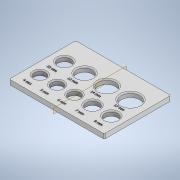
# Autodesk Inventor part: mmHexSocketSetOf9
Saved by Autodesk Inventor 2020.3 (Build 243373000, 373)
## iProperties
Created: 2020-03-13
Part Number: mmHexSocketSetOf9
Material: Generic
Document SubType Name: Modeling
Designer: robst
Density: 1 g/cm^3
Appearance: Default
Author: robst
Autodesk Inventor part; units mm, degrees
(part 1 of 2)
ref_plane "XZ Plane" through (0, 0, 0) normal (0, 1, 0) x (-1, 0, 0)
ref_plane "XY Plane" through (0, 0, 0) normal (0, 0, 1) x (1, 0, 0)
sketch "Sketch1" plane through (0, 0, 0) normal (0, 1, 0) x (-1, 0, 0)
  line L0 (63.5, 44.45) -> (-63.5, 44.45)
  line L1 (-63.5, 44.45) -> (-63.5, -44.45)
  line L2 (-63.5, -44.45) -> (63.5, -44.45)
  line L3 (63.5, -44.45) -> (63.5, 44.45)
  line L4 (63.5, 44.45) -> (-63.5, -44.45) construction
  line L5 (-63.5, 44.45) -> (63.5, -44.45) construction
  point P0 (0, 0)
  dimension "d3" = 88.9
  dimension "d13" = 127
  constraints: 12 end point, 2 midpoint, 2 parallel, 1 horizontal, 1 perpendicular
  measures "d3" distance of L2.end L0.start
  measures "d13" distance of L1.end L2.end
extrude "Extrusion1" add sketch "Sketch1" against normal blind 6.35
sketch "Sketch4" plane through (0, 0, 0) normal (0, 1, 0) x (1, 0, 0)
  line L0 (-63.5, -44.45) -> (-63.5, 44.45) construction
  line L1 (-63.5, -19.05) -> (63.5, -19.05) construction
  line L2 (63.5, 44.45) -> (63.5, -44.45) construction
  line L3 (-63.5, -44.45) -> (63.5, -44.45) projected
  circle A0 centre (-47.9975, -19.05) radius 7.62
  circle A1 centre (-24.8751, -19.05) radius 7.62
  circle A2 centre (-1.7526, -19.05) radius 7.62
  circle A3 centre (22.3859, -19.05) radius 8.636
  circle A4 centre (47.5403, -19.05) radius 8.636
  line L4 (-63.5, 12.7) -> (63.5, 12.7) construction
  circle A5 centre (-46.99, 12.7) radius 8.636
  circle A6 centre (-20.0025, 12.7) radius 10.4775
  circle A7 centre (9.779, 12.7) radius 11.43
  circle A8 centre (41.4655, 12.7) radius 12.3825
  point P0 (0, 0)
  dimension "d16" = 25.4
  dimension "hex4mmHole" = 15.24
  dimension "gap0" = 7.8825
  dimension "hex5mmHole" = 15.24
  dimension "gap1" = 23.1225
  dimension "hex6mmHole" = 15.24
  dimension "gap2" = 23.1225
  dimension "gap3" = 24.1385
  dimension "gap4" = 25.1545
  dimension "hex7mmHole" = 17.272
  dimension "hex8mmHole" = 17.272
  dimension "d27" = 7.3237
  dimension "frontToBackRowGap" = 31.75
  dimension "gap5" = 7.874
  dimension "hex10mmHole" = 17.272
  dimension "hex12mmHole" = 20.955
  dimension "gap6" = 26.9875
  dimension "hex14mmHole" = 22.86
  dimension "gap7" = 29.7815
  dimension "hex17mmHole" = 24.765
  dimension "gap8" = 31.6865
  dimension "d37" = 9.652
  constraints: 13 point on line, 9 centre point, 4 end point, 1 horizontal, 1 perpendicular
  measures "d16" distance between parallel lines of L1 L3
  measures "hex4mmHole" diameter of A0
  measures "gap0" distance edge to line of A0 L0
  measures "hex5mmHole" diameter of A1
  measures "gap1" distance of A1.centre A0.centre
  measures "hex6mmHole" diameter of A2
  measures "gap2" distance of A2.centre A1.centre
  measures "gap3" distance of A3.centre A2.centre
  measures "gap4" distance of A4.centre A3.centre
  measures "hex7mmHole" diameter of A3
  measures "hex8mmHole" diameter of A4
  measures "d27" distance edge to line of A4 L2
  measures "frontToBackRowGap" distance between parallel lines of L4 L1
  measures "gap5" distance edge to line of A5 L0
  measures "hex10mmHole" diameter of A5
  measures "hex12mmHole" diameter of A6
  measures "gap6" distance of A6.centre A5.centre
  measures "hex14mmHole" diameter of A7
  measures "gap7" distance of A7.centre A6.centre
  measures "hex17mmHole" diameter of A8
  measures "gap8" distance of A8.centre A7.centre
  measures "d37" distance edge to line of A8 L2
extrude "Extrusion3" cut sketch "Sketch4" against normal through all
sketch "Sketch7" plane through (0, 0, 0) normal (0, 1, 0) x (1, 0, 0)
  circle A0 centre (-47.9975, -19.05) radius 7.62 construction
  line L0 (63.5, -44.45) -> (-63.5, -44.45) construction
  line L1 (-55.6175, -35.6779) -> (-40.3775, -35.6779) construction
  line L2 (-32.4951, -35.6779) -> (-17.2551, -35.6779) construction
  line L3 (-9.3726, -35.6779) -> (5.8674, -35.6779) construction
  line L4 (13.7499, -35.6779) -> (30.7679, -35.6779) construction
  line L5 (38.6503, -35.6779) -> (55.6683, -35.6779) construction
  line L6 (-55.626, -3.81) -> (-38.354, -3.81) construction
  line L7 (-30.48, -3.81) -> (-7.62, -3.81) construction
  line L8 (0.254, -3.81) -> (23.114, -3.81) construction
  line L9 (30.988, -3.81) -> (55.626, -3.81) construction
  line L10 (-51.5027, -5.334) -> (-52.9897, -5.334)
  line L11 (-52.9897, -5.334) -> (-52.9897, -5.0228)
  line L12 (-52.9897, -5.0228) -> (-52.4364, -5.0228)
  line L13 (-52.4364, -5.0228) -> (-52.4364, -2.9801)
  line L14 (-52.4364, -2.9801) -> (-52.9897, -2.9801)
  line L15 (-52.9897, -2.9801) -> (-52.9897, -2.701)
  spline S0 degree 2 poles (-52.9897, -2.701) (-52.676, -2.701) (-52.3796, -2.5231) (-52.3598, -2.2761) knots 0 0 0 1 2 2 2
  line L16 (-52.3598, -2.2761) -> (-52.0437, -2.2761)
  line L17 (-52.0437, -2.2761) -> (-52.0437, -5.0228)
  line L18 (-52.0437, -5.0228) -> (-51.5027, -5.0228)
  line L19 (-51.5027, -5.0228) -> (-51.5027, -5.334)
  spline S1 degree 2 poles (-49.0451, -3.81) (-49.0451, -4.63) (-49.5218, -5.3982) (-50.0182, -5.3982) knots 0 0 0 1 2 2 2
  spline S2 degree 2 poles (-50.0182, -5.3982) (-50.5221, -5.3982) (-50.9939, -4.6152) (-50.9939, -3.8125) knots 0 0 0 1 2 2 2
  spline S3 degree 2 poles (-50.9939, -3.8125) (-50.9939, -2.9875) (-50.5172, -2.2242) (-50.0182, -2.2242) knots 0 0 0 1 2 2 2
  spline S4 degree 2 poles (-50.0182, -2.2242) (-49.5168, -2.2242) (-49.0451, -3.0147) (-49.0451, -3.81) knots 0 0 0 1 2 2 2
  spline S5 degree 2 poles (-49.5687, -4.7387) (-49.5094, -4.5881) (-49.46, -4.1237) (-49.46, -3.81) knots 0 0 0 1 2 2 2
  spline S6 degree 2 poles (-49.46, -3.81) (-49.46, -3.4963) (-49.5094, -3.0344) (-49.5712, -2.8788) knots 0 0 0 1 2 2 2
  spline S7 degree 2 poles (-49.5712, -2.8788) (-49.6329, -2.7232) (-49.8478, -2.5626) (-50.0182, -2.5626) knots 0 0 0 1 2 2 2
  spline S8 degree 2 poles (-50.0182, -2.5626) (-50.1887, -2.5626) (-50.4085, -2.7232) (-50.4727, -2.8837) knots 0 0 0 1 2 2 2
  spline S9 degree 2 poles (-50.4727, -2.8837) (-50.5345, -3.0394) (-50.5789, -3.5136) (-50.5789, -3.8125) knots 0 0 0 1 2 2 2
  spline S10 degree 2 poles (-50.5789, -3.8125) (-50.5789, -4.1336) (-50.5394, -4.5634) (-50.4752, -4.7313) knots 0 0 0 1 2 2 2
  spline S11 degree 2 poles (-50.4752, -4.7313) (-50.4159, -4.8894) (-50.1961, -5.0598) (-50.0182, -5.0598) knots 0 0 0 1 2 2 2
  spline S12 degree 2 poles (-50.0182, -5.0598) (-49.8503, -5.0598) (-49.6304, -4.8993) (-49.5687, -4.7387) knots 0 0 0 1 2 2 2
  line L20 (-44.6954, -5.334) -> (-44.6954, -4.0101)
  spline S13 degree 2 poles (-44.6954, -4.0101) (-44.6954, -3.852) (-44.7201, -3.5828) (-44.7596, -3.5087) knots 0 0 0 1 2 2 2
  spline S14 degree 2 poles (-44.7596, -3.5087) (-44.7991, -3.4271) (-44.9498, -3.3481) (-45.0807, -3.3481) knots 0 0 0 1 2 2 2
  spline S15 degree 2 poles (-45.0807, -3.3481) (-45.1992, -3.3481) (-45.4709, -3.4938) (-45.6142, -3.6322) knots 0 0 0 1 2 2 2
  spline S16 degree 2 poles (-45.6142, -3.6322) (-45.6117, -3.6667) (-45.6068, -3.7631) (-45.6068, -3.8273) knots 0 0 0 1 2 2 2
  line L21 (-45.6068, -3.8273) -> (-45.6068, -5.334)
  line L22 (-45.6068, -5.334) -> (-45.9921, -5.334)
  line L23 (-45.9921, -5.334) -> (-45.9921, -4.0101)
  spline S17 degree 2 poles (-45.9921, -4.0101) (-45.9921, -3.852) (-46.0168, -3.5828) (-46.0563, -3.5087) knots 0 0 0 1 2 2 2
  spline S18 degree 2 poles (-46.0563, -3.5087) (-46.0959, -3.4271) (-46.2465, -3.3481) (-46.3774, -3.3481) knots 0 0 0 1 2 2 2
  spline S19 degree 2 poles (-46.3774, -3.3481) (-46.5009, -3.3481) (-46.7751, -3.5037) (-46.9035, -3.6247) knots 0 0 0 1 2 2 2
  line L24 (-46.9035, -3.6247) -> (-46.9035, -5.334)
  line L25 (-46.9035, -5.334) -> (-47.2889, -5.334)
  line L26 (-47.2889, -5.334) -> (-47.2889, -3.0468)
  line L27 (-47.2889, -3.0468) -> (-46.9035, -3.0468)
  line L28 (-46.9035, -3.0468) -> (-46.9035, -3.2987)
  spline S20 degree 2 poles (-46.9035, -3.2987) (-46.7529, -3.148) (-46.4565, -2.9825) (-46.2786, -2.9825) knots 0 0 0 1 2 2 2
  spline S21 degree 2 poles (-46.2786, -2.9825) (-46.0761, -2.9825) (-45.7624, -3.1678) (-45.6809, -3.3777) knots 0 0 0 1 2 2 2
  spline S22 degree 2 poles (-45.6809, -3.3777) (-45.5055, -3.1826) (-45.1745, -2.9825) (-44.9819, -2.9825) knots 0 0 0 1 2 2 2
  spline S23 degree 2 poles (-44.9819, -2.9825) (-44.8337, -2.9825) (-44.5916, -3.0739) (-44.5027, -3.1777) knots 0 0 0 1 2 2 2
  spline S24 degree 2 poles (-44.5027, -3.1777) (-44.4113, -3.2814) (-44.31, -3.5926) (-44.31, -3.8273) knots 0 0 0 1 2 2 2
  line L29 (-44.31, -3.8273) -> (-44.31, -5.334)
  line L30 (-44.31, -5.334) -> (-44.6954, -5.334)
  line L31 (-41.1756, -5.334) -> (-41.1756, -4.0101)
  spline S25 degree 2 poles (-41.1756, -4.0101) (-41.1756, -3.852) (-41.2003, -3.5828) (-41.2398, -3.5087) knots 0 0 0 1 2 2 2
  spline S26 degree 2 poles (-41.2398, -3.5087) (-41.2793, -3.4271) (-41.43, -3.3481) (-41.5609, -3.3481) knots 0 0 0 1 2 2 2
  spline S27 degree 2 poles (-41.5609, -3.3481) (-41.6795, -3.3481) (-41.9512, -3.4938) (-42.0944, -3.6322) knots 0 0 0 1 2 2 2
  spline S28 degree 2 poles (-42.0944, -3.6322) (-42.092, -3.6667) (-42.087, -3.7631) (-42.087, -3.8273) knots 0 0 0 1 2 2 2
  line L32 (-42.087, -3.8273) -> (-42.087, -5.334)
  line L33 (-42.087, -5.334) -> (-42.4723, -5.334)
  line L34 (-42.4723, -5.334) -> (-42.4723, -4.0101)
  spline S29 degree 2 poles (-42.4723, -4.0101) (-42.4723, -3.852) (-42.497, -3.5828) (-42.5366, -3.5087) knots 0 0 0 1 2 2 2
  spline S30 degree 2 poles (-42.5366, -3.5087) (-42.5761, -3.4271) (-42.7268, -3.3481) (-42.8577, -3.3481) knots 0 0 0 1 2 2 2
  spline S31 degree 2 poles (-42.8577, -3.3481) (-42.9812, -3.3481) (-43.2553, -3.5037) (-43.3838, -3.6247) knots 0 0 0 1 2 2 2
  line L35 (-43.3838, -3.6247) -> (-43.3838, -5.334)
  line L36 (-43.3838, -5.334) -> (-43.7691, -5.334)
  line L37 (-43.7691, -5.334) -> (-43.7691, -3.0468)
  line L38 (-43.7691, -3.0468) -> (-43.3838, -3.0468)
  line L39 (-43.3838, -3.0468) -> (-43.3838, -3.2987)
  spline S32 degree 2 poles (-43.3838, -3.2987) (-43.2331, -3.148) (-42.9367, -2.9825) (-42.7589, -2.9825) knots 0 0 0 1 2 2 2
  spline S33 degree 2 poles (-42.7589, -2.9825) (-42.5563, -2.9825) (-42.2426, -3.1678) (-42.1611, -3.3777) knots 0 0 0 1 2 2 2
  spline S34 degree 2 poles (-42.1611, -3.3777) (-41.9857, -3.1826) (-41.6548, -2.9825) (-41.4621, -2.9825) knots 0 0 0 1 2 2 2
  spline S35 degree 2 poles (-41.4621, -2.9825) (-41.3139, -2.9825) (-41.0718, -3.0739) (-40.9829, -3.1777) knots 0 0 0 1 2 2 2
  spline S36 degree 2 poles (-40.9829, -3.1777) (-40.8915, -3.2814) (-40.7903, -3.5926) (-40.7903, -3.8273) knots 0 0 0 1 2 2 2
  line L40 (-40.7903, -3.8273) -> (-40.7903, -5.334)
  line L41 (-40.7903, -5.334) -> (-41.1756, -5.334)
  line L42 (-23.5627, -5.334) -> (-25.0497, -5.334)
  line L43 (-25.0497, -5.334) -> (-25.0497, -5.0228)
  line L44 (-25.0497, -5.0228) -> (-24.4964, -5.0228)
  line L45 (-24.4964, -5.0228) -> (-24.4964, -2.9801)
  line L46 (-24.4964, -2.9801) -> (-25.0497, -2.9801)
  line L47 (-25.0497, -2.9801) -> (-25.0497, -2.701)
  spline S37 degree 2 poles (-25.0497, -2.701) (-24.736, -2.701) (-24.4396, -2.5231) (-24.4198, -2.2761) knots 0 0 0 1 2 2 2
  line L48 (-24.4198, -2.2761) -> (-24.1037, -2.2761)
  line L49 (-24.1037, -2.2761) -> (-24.1037, -5.0228)
  line L50 (-24.1037, -5.0228) -> (-23.5627, -5.0228)
  line L51 (-23.5627, -5.0228) -> (-23.5627, -5.334)
  line L52 (-21.1223, -5.334) -> (-23.002, -5.334)
  line L53 (-23.002, -5.334) -> (-23.002, -4.9017)
  spline S38 degree 2 poles (-23.002, -4.9017) (-22.7995, -4.7116) (-22.4389, -4.3583) (-22.266, -4.1682) knots 0 0 0 1 2 2 2
  spline S39 degree 2 poles (-22.266, -4.1682) (-21.9177, -3.7853) (-21.6633, -3.3259) (-21.6633, -3.0813) knots 0 0 0 1 2 2 2
  spline S40 degree 2 poles (-21.6633, -3.0813) (-21.6633, -2.9529) (-21.7423, -2.7602) (-21.8139, -2.6985) knots 0 0 0 1 2 2 2
  spline S41 degree 2 poles (-21.8139, -2.6985) (-21.8856, -2.6367) (-22.0733, -2.575) (-22.1869, -2.575) knots 0 0 0 1 2 2 2
  spline S42 degree 2 poles (-22.1869, -2.575) (-22.2956, -2.575) (-22.5179, -2.6293) (-22.6192, -2.6713) knots 0 0 0 1 2 2 2
  spline S43 degree 2 poles (-22.6192, -2.6713) (-22.7056, -2.7059) (-22.8662, -2.8047) (-22.9156, -2.8393) knots 0 0 0 1 2 2 2
  line L54 (-22.9156, -2.8393) -> (-22.9378, -2.8393)
  line L55 (-22.9378, -2.8393) -> (-22.9378, -2.4046)
  spline S44 degree 2 poles (-22.9378, -2.4046) (-22.8118, -2.3428) (-22.3598, -2.2218) (-22.1573, -2.2218) knots 0 0 0 1 2 2 2
  spline S45 degree 2 poles (-22.1573, -2.2218) (-21.73, -2.2218) (-21.2483, -2.6738) (-21.2483, -3.0591) knots 0 0 0 1 2 2 2
  spline S46 degree 2 poles (-21.2483, -3.0591) (-21.2483, -3.2394) (-21.3323, -3.5408) (-21.4064, -3.6692) knots 0 0 0 1 2 2 2
  spline S47 degree 2 poles (-21.4064, -3.6692) (-21.4805, -3.8026) (-21.6954, -4.0644) (-21.8139, -4.1904) knots 0 0 0 1 2 2 2
  spline S48 degree 2 poles (-21.8139, -4.1904) (-22.0066, -4.4003) (-22.4784, -4.8499) (-22.6192, -4.9808) knots 0 0 0 1 2 2 2
  line L56 (-22.6192, -4.9808) -> (-21.1223, -4.9808)
  line L57 (-21.1223, -4.9808) -> (-21.1223, -5.334)
  line L58 (-16.7554, -5.334) -> (-16.7554, -4.0101)
  spline S49 degree 2 poles (-16.7554, -4.0101) (-16.7554, -3.852) (-16.7801, -3.5828) (-16.8196, -3.5087) knots 0 0 0 1 2 2 2
  spline S50 degree 2 poles (-16.8196, -3.5087) (-16.8591, -3.4271) (-17.0098, -3.3481) (-17.1407, -3.3481) knots 0 0 0 1 2 2 2
  spline S51 degree 2 poles (-17.1407, -3.3481) (-17.2592, -3.3481) (-17.5309, -3.4938) (-17.6742, -3.6322) knots 0 0 0 1 2 2 2
  spline S52 degree 2 poles (-17.6742, -3.6322) (-17.6717, -3.6667) (-17.6668, -3.7631) (-17.6668, -3.8273) knots 0 0 0 1 2 2 2
  line L59 (-17.6668, -3.8273) -> (-17.6668, -5.334)
  line L60 (-17.6668, -5.334) -> (-18.0521, -5.334)
  line L61 (-18.0521, -5.334) -> (-18.0521, -4.0101)
  spline S53 degree 2 poles (-18.0521, -4.0101) (-18.0521, -3.852) (-18.0768, -3.5828) (-18.1163, -3.5087) knots 0 0 0 1 2 2 2
  spline S54 degree 2 poles (-18.1163, -3.5087) (-18.1559, -3.4271) (-18.3065, -3.3481) (-18.4374, -3.3481) knots 0 0 0 1 2 2 2
  spline S55 degree 2 poles (-18.4374, -3.3481) (-18.5609, -3.3481) (-18.8351, -3.5037) (-18.9635, -3.6247) knots 0 0 0 1 2 2 2
  line L62 (-18.9635, -3.6247) -> (-18.9635, -5.334)
  line L63 (-18.9635, -5.334) -> (-19.3489, -5.334)
  line L64 (-19.3489, -5.334) -> (-19.3489, -3.0468)
  line L65 (-19.3489, -3.0468) -> (-18.9635, -3.0468)
  line L66 (-18.9635, -3.0468) -> (-18.9635, -3.2987)
  spline S56 degree 2 poles (-18.9635, -3.2987) (-18.8129, -3.148) (-18.5165, -2.9825) (-18.3386, -2.9825) knots 0 0 0 1 2 2 2
  spline S57 degree 2 poles (-18.3386, -2.9825) (-18.1361, -2.9825) (-17.8224, -3.1678) (-17.7409, -3.3777) knots 0 0 0 1 2 2 2
  spline S58 degree 2 poles (-17.7409, -3.3777) (-17.5655, -3.1826) (-17.2345, -2.9825) (-17.0419, -2.9825) knots 0 0 0 1 2 2 2
  spline S59 degree 2 poles (-17.0419, -2.9825) (-16.8937, -2.9825) (-16.6516, -3.0739) (-16.5627, -3.1777) knots 0 0 0 1 2 2 2
  spline S60 degree 2 poles (-16.5627, -3.1777) (-16.4713, -3.2814) (-16.37, -3.5926) (-16.37, -3.8273) knots 0 0 0 1 2 2 2
  line L67 (-16.37, -3.8273) -> (-16.37, -5.334)
  line L68 (-16.37, -5.334) -> (-16.7554, -5.334)
  line L69 (-13.2356, -5.334) -> (-13.2356, -4.0101)
  spline S61 degree 2 poles (-13.2356, -4.0101) (-13.2356, -3.852) (-13.2603, -3.5828) (-13.2998, -3.5087) knots 0 0 0 1 2 2 2
  spline S62 degree 2 poles (-13.2998, -3.5087) (-13.3393, -3.4271) (-13.49, -3.3481) (-13.6209, -3.3481) knots 0 0 0 1 2 2 2
  spline S63 degree 2 poles (-13.6209, -3.3481) (-13.7395, -3.3481) (-14.0112, -3.4938) (-14.1544, -3.6322) knots 0 0 0 1 2 2 2
  spline S64 degree 2 poles (-14.1544, -3.6322) (-14.152, -3.6667) (-14.147, -3.7631) (-14.147, -3.8273) knots 0 0 0 1 2 2 2
  line L70 (-14.147, -3.8273) -> (-14.147, -5.334)
  line L71 (-14.147, -5.334) -> (-14.5323, -5.334)
  line L72 (-14.5323, -5.334) -> (-14.5323, -4.0101)
  spline S65 degree 2 poles (-14.5323, -4.0101) (-14.5323, -3.852) (-14.557, -3.5828) (-14.5966, -3.5087) knots 0 0 0 1 2 2 2
  spline S66 degree 2 poles (-14.5966, -3.5087) (-14.6361, -3.4271) (-14.7868, -3.3481) (-14.9177, -3.3481) knots 0 0 0 1 2 2 2
  spline S67 degree 2 poles (-14.9177, -3.3481) (-15.0412, -3.3481) (-15.3153, -3.5037) (-15.4438, -3.6247) knots 0 0 0 1 2 2 2
  line L73 (-15.4438, -3.6247) -> (-15.4438, -5.334)
  line L74 (-15.4438, -5.334) -> (-15.8291, -5.334)
  line L75 (-15.8291, -5.334) -> (-15.8291, -3.0468)
  line L76 (-15.8291, -3.0468) -> (-15.4438, -3.0468)
  line L77 (-15.4438, -3.0468) -> (-15.4438, -3.2987)
  spline S68 degree 2 poles (-15.4438, -3.2987) (-15.2931, -3.148) (-14.9967, -2.9825) (-14.8189, -2.9825) knots 0 0 0 1 2 2 2
  spline S69 degree 2 poles (-14.8189, -2.9825) (-14.6163, -2.9825) (-14.3026, -3.1678) (-14.2211, -3.3777) knots 0 0 0 1 2 2 2
  spline S70 degree 2 poles (-14.2211, -3.3777) (-14.0457, -3.1826) (-13.7148, -2.9825) (-13.5221, -2.9825) knots 0 0 0 1 2 2 2
  spline S71 degree 2 poles (-13.5221, -2.9825) (-13.3739, -2.9825) (-13.1318, -3.0739) (-13.0429, -3.1777) knots 0 0 0 1 2 2 2
  spline S72 degree 2 poles (-13.0429, -3.1777) (-12.9515, -3.2814) (-12.8503, -3.5926) (-12.8503, -3.8273) knots 0 0 0 1 2 2 2
  line L78 (-12.8503, -3.8273) -> (-12.8503, -5.334)
  line L79 (-12.8503, -5.334) -> (-13.2356, -5.334)
  line L80 (7.1713, -5.334) -> (5.6843, -5.334)
  line L81 (5.6843, -5.334) -> (5.6843, -5.0228)
  line L82 (5.6843, -5.0228) -> (6.2376, -5.0228)
  line L83 (6.2376, -5.0228) -> (6.2376, -2.9801)
  line L84 (6.2376, -2.9801) -> (5.6843, -2.9801)
  line L85 (5.6843, -2.9801) -> (5.6843, -2.701)
  spline S73 degree 2 poles (5.6843, -2.701) (5.998, -2.701) (6.2944, -2.5231) (6.3142, -2.2761) knots 0 0 0 1 2 2 2
  line L86 (6.3142, -2.2761) -> (6.6303, -2.2761)
  line L87 (6.6303, -2.2761) -> (6.6303, -5.0228)
  line L88 (6.6303, -5.0228) -> (7.1713, -5.0228)
  line L89 (7.1713, -5.0228) -> (7.1713, -5.334)
  line L90 (9.6932, -4.2867) -> (9.3301, -4.2867)
  line L91 (9.3301, -4.2867) -> (9.3301, -5.334)
  line L92 (9.3301, -5.334) -> (8.9373, -5.334)
  line L93 (8.9373, -5.334) -> (8.9373, -4.2867)
  line L94 (8.9373, -4.2867) -> (7.5912, -4.2867)
  line L95 (7.5912, -4.2867) -> (7.5912, -3.8569)
  line L96 (7.5912, -3.8569) -> (8.9546, -2.286)
  line L97 (8.9546, -2.286) -> (9.3301, -2.286)
  line L98 (9.3301, -2.286) -> (9.3301, -3.9582)
  line L99 (9.3301, -3.9582) -> (9.6932, -3.9582)
  line L100 (9.6932, -3.9582) -> (9.6932, -4.2867)
  line L101 (8.9373, -3.9582) -> (8.9373, -2.7677)
  line L102 (8.9373, -2.7677) -> (7.9123, -3.9582)
  line L103 (7.9123, -3.9582) -> (8.9373, -3.9582)
  line L104 (13.9786, -5.334) -> (13.9786, -4.0101)
  spline S74 degree 2 poles (13.9786, -4.0101) (13.9786, -3.852) (13.9539, -3.5828) (13.9144, -3.5087) knots 0 0 0 1 2 2 2
  spline S75 degree 2 poles (13.9144, -3.5087) (13.8749, -3.4271) (13.7242, -3.3481) (13.5933, -3.3481) knots 0 0 0 1 2 2 2
  spline S76 degree 2 poles (13.5933, -3.3481) (13.4748, -3.3481) (13.2031, -3.4938) (13.0598, -3.6322) knots 0 0 0 1 2 2 2
  spline S77 degree 2 poles (13.0598, -3.6322) (13.0623, -3.6667) (13.0672, -3.7631) (13.0672, -3.8273) knots 0 0 0 1 2 2 2
  line L105 (13.0672, -3.8273) -> (13.0672, -5.334)
  line L106 (13.0672, -5.334) -> (12.6819, -5.334)
  line L107 (12.6819, -5.334) -> (12.6819, -4.0101)
  spline S78 degree 2 poles (12.6819, -4.0101) (12.6819, -3.852) (12.6572, -3.5828) (12.6177, -3.5087) knots 0 0 0 1 2 2 2
  spline S79 degree 2 poles (12.6177, -3.5087) (12.5781, -3.4271) (12.4275, -3.3481) (12.2966, -3.3481) knots 0 0 0 1 2 2 2
  spline S80 degree 2 poles (12.2966, -3.3481) (12.1731, -3.3481) (11.8989, -3.5037) (11.7705, -3.6247) knots 0 0 0 1 2 2 2
  line L108 (11.7705, -3.6247) -> (11.7705, -5.334)
  line L109 (11.7705, -5.334) -> (11.3851, -5.334)
  line L110 (11.3851, -5.334) -> (11.3851, -3.0468)
  line L111 (11.3851, -3.0468) -> (11.7705, -3.0468)
  line L112 (11.7705, -3.0468) -> (11.7705, -3.2987)
  spline S81 degree 2 poles (11.7705, -3.2987) (11.9211, -3.148) (12.2175, -2.9825) (12.3954, -2.9825) knots 0 0 0 1 2 2 2
  spline S82 degree 2 poles (12.3954, -2.9825) (12.5979, -2.9825) (12.9116, -3.1678) (12.9931, -3.3777) knots 0 0 0 1 2 2 2
  spline S83 degree 2 poles (12.9931, -3.3777) (13.1685, -3.1826) (13.4995, -2.9825) (13.6921, -2.9825) knots 0 0 0 1 2 2 2
  spline S84 degree 2 poles (13.6921, -2.9825) (13.8403, -2.9825) (14.0824, -3.0739) (14.1713, -3.1777) knots 0 0 0 1 2 2 2
  spline S85 degree 2 poles (14.1713, -3.1777) (14.2627, -3.2814) (14.364, -3.5926) (14.364, -3.8273) knots 0 0 0 1 2 2 2
  line L113 (14.364, -3.8273) -> (14.364, -5.334)
  line L114 (14.364, -5.334) -> (13.9786, -5.334)
  line L115 (17.4984, -5.334) -> (17.4984, -4.0101)
  spline S86 degree 2 poles (17.4984, -4.0101) (17.4984, -3.852) (17.4737, -3.5828) (17.4342, -3.5087) knots 0 0 0 1 2 2 2
  spline S87 degree 2 poles (17.4342, -3.5087) (17.3947, -3.4271) (17.244, -3.3481) (17.1131, -3.3481) knots 0 0 0 1 2 2 2
  spline S88 degree 2 poles (17.1131, -3.3481) (16.9945, -3.3481) (16.7228, -3.4938) (16.5796, -3.6322) knots 0 0 0 1 2 2 2
  spline S89 degree 2 poles (16.5796, -3.6322) (16.582, -3.6667) (16.587, -3.7631) (16.587, -3.8273) knots 0 0 0 1 2 2 2
  line L116 (16.587, -3.8273) -> (16.587, -5.334)
  line L117 (16.587, -5.334) -> (16.2017, -5.334)
  line L118 (16.2017, -5.334) -> (16.2017, -4.0101)
  spline S90 degree 2 poles (16.2017, -4.0101) (16.2017, -3.852) (16.177, -3.5828) (16.1374, -3.5087) knots 0 0 0 1 2 2 2
  spline S91 degree 2 poles (16.1374, -3.5087) (16.0979, -3.4271) (15.9472, -3.3481) (15.8163, -3.3481) knots 0 0 0 1 2 2 2
  spline S92 degree 2 poles (15.8163, -3.3481) (15.6928, -3.3481) (15.4187, -3.5037) (15.2902, -3.6247) knots 0 0 0 1 2 2 2
  line L119 (15.2902, -3.6247) -> (15.2902, -5.334)
  line L120 (15.2902, -5.334) -> (14.9049, -5.334)
  line L121 (14.9049, -5.334) -> (14.9049, -3.0468)
  line L122 (14.9049, -3.0468) -> (15.2902, -3.0468)
  line L123 (15.2902, -3.0468) -> (15.2902, -3.2987)
  spline S93 degree 2 poles (15.2902, -3.2987) (15.4409, -3.148) (15.7373, -2.9825) (15.9151, -2.9825) knots 0 0 0 1 2 2 2
  spline S94 degree 2 poles (15.9151, -2.9825) (16.1177, -2.9825) (16.4314, -3.1678) (16.5129, -3.3777) knots 0 0 0 1 2 2 2
  spline S95 degree 2 poles (16.5129, -3.3777) (16.6883, -3.1826) (17.0192, -2.9825) (17.2119, -2.9825) knots 0 0 0 1 2 2 2
  spline S96 degree 2 poles (17.2119, -2.9825) (17.3601, -2.9825) (17.6022, -3.0739) (17.6911, -3.1777) knots 0 0 0 1 2 2 2
  spline S97 degree 2 poles (17.6911, -3.1777) (17.7825, -3.2814) (17.8837, -3.5926) (17.8837, -3.8273) knots 0 0 0 1 2 2 2
  line L124 (17.8837, -3.8273) -> (17.8837, -5.334)
  line L125 (17.8837, -5.334) -> (17.4984, -5.334)
  line L126 (38.7943, -5.334) -> (37.3073, -5.334)
  line L127 (37.3073, -5.334) -> (37.3073, -5.0228)
  line L128 (37.3073, -5.0228) -> (37.8606, -5.0228)
  line L129 (37.8606, -5.0228) -> (37.8606, -2.9801)
  line L130 (37.8606, -2.9801) -> (37.3073, -2.9801)
  line L131 (37.3073, -2.9801) -> (37.3073, -2.701)
  spline S98 degree 2 poles (37.3073, -2.701) (37.621, -2.701) (37.9174, -2.5231) (37.9372, -2.2761) knots 0 0 0 1 2 2 2
  line L132 (37.9372, -2.2761) -> (38.2533, -2.2761)
  line L133 (38.2533, -2.2761) -> (38.2533, -5.0228)
  line L134 (38.2533, -5.0228) -> (38.7943, -5.0228)
  line L135 (38.7943, -5.0228) -> (38.7943, -5.334)
  line L136 (41.2692, -2.743) -> (39.9502, -5.334)
  line L137 (39.9502, -5.334) -> (39.5155, -5.334)
  line L138 (39.5155, -5.334) -> (40.9086, -2.6442)
  line L139 (40.9086, -2.6442) -> (39.3352, -2.6442)
  line L140 (39.3352, -2.6442) -> (39.3352, -2.286)
  line L141 (39.3352, -2.286) -> (41.2692, -2.286)
  line L142 (41.2692, -2.286) -> (41.2692, -2.743)
  line L143 (45.6016, -5.334) -> (45.6016, -4.0101)
  spline S99 degree 2 poles (45.6016, -4.0101) (45.6016, -3.852) (45.5769, -3.5828) (45.5374, -3.5087) knots 0 0 0 1 2 2 2
  spline S100 degree 2 poles (45.5374, -3.5087) (45.4979, -3.4271) (45.3472, -3.3481) (45.2163, -3.3481) knots 0 0 0 1 2 2 2
  spline S101 degree 2 poles (45.2163, -3.3481) (45.0978, -3.3481) (44.8261, -3.4938) (44.6828, -3.6322) knots 0 0 0 1 2 2 2
  spline S102 degree 2 poles (44.6828, -3.6322) (44.6853, -3.6667) (44.6902, -3.7631) (44.6902, -3.8273) knots 0 0 0 1 2 2 2
  line L144 (44.6902, -3.8273) -> (44.6902, -5.334)
  line L145 (44.6902, -5.334) -> (44.3049, -5.334)
  line L146 (44.3049, -5.334) -> (44.3049, -4.0101)
  spline S103 degree 2 poles (44.3049, -4.0101) (44.3049, -3.852) (44.2802, -3.5828) (44.2407, -3.5087) knots 0 0 0 1 2 2 2
  spline S104 degree 2 poles (44.2407, -3.5087) (44.2011, -3.4271) (44.0505, -3.3481) (43.9196, -3.3481) knots 0 0 0 1 2 2 2
  spline S105 degree 2 poles (43.9196, -3.3481) (43.7961, -3.3481) (43.5219, -3.5037) (43.3935, -3.6247) knots 0 0 0 1 2 2 2
  line L147 (43.3935, -3.6247) -> (43.3935, -5.334)
  line L148 (43.3935, -5.334) -> (43.0081, -5.334)
  line L149 (43.0081, -5.334) -> (43.0081, -3.0468)
  line L150 (43.0081, -3.0468) -> (43.3935, -3.0468)
  line L151 (43.3935, -3.0468) -> (43.3935, -3.2987)
  spline S106 degree 2 poles (43.3935, -3.2987) (43.5441, -3.148) (43.8405, -2.9825) (44.0184, -2.9825) knots 0 0 0 1 2 2 2
  spline S107 degree 2 poles (44.0184, -2.9825) (44.2209, -2.9825) (44.5346, -3.1678) (44.6161, -3.3777) knots 0 0 0 1 2 2 2
  spline S108 degree 2 poles (44.6161, -3.3777) (44.7915, -3.1826) (45.1225, -2.9825) (45.3151, -2.9825) knots 0 0 0 1 2 2 2
  spline S109 degree 2 poles (45.3151, -2.9825) (45.4633, -2.9825) (45.7054, -3.0739) (45.7943, -3.1777) knots 0 0 0 1 2 2 2
  spline S110 degree 2 poles (45.7943, -3.1777) (45.8857, -3.2814) (45.987, -3.5926) (45.987, -3.8273) knots 0 0 0 1 2 2 2
  line L152 (45.987, -3.8273) -> (45.987, -5.334)
  line L153 (45.987, -5.334) -> (45.6016, -5.334)
  line L154 (49.1214, -5.334) -> (49.1214, -4.0101)
  spline S111 degree 2 poles (49.1214, -4.0101) (49.1214, -3.852) (49.0967, -3.5828) (49.0572, -3.5087) knots 0 0 0 1 2 2 2
  spline S112 degree 2 poles (49.0572, -3.5087) (49.0177, -3.4271) (48.867, -3.3481) (48.7361, -3.3481) knots 0 0 0 1 2 2 2
  spline S113 degree 2 poles (48.7361, -3.3481) (48.6175, -3.3481) (48.3458, -3.4938) (48.2026, -3.6322) knots 0 0 0 1 2 2 2
  spline S114 degree 2 poles (48.2026, -3.6322) (48.205, -3.6667) (48.21, -3.7631) (48.21, -3.8273) knots 0 0 0 1 2 2 2
  line L155 (48.21, -3.8273) -> (48.21, -5.334)
  line L156 (48.21, -5.334) -> (47.8247, -5.334)
  line L157 (47.8247, -5.334) -> (47.8247, -4.0101)
  spline S115 degree 2 poles (47.8247, -4.0101) (47.8247, -3.852) (47.8, -3.5828) (47.7604, -3.5087) knots 0 0 0 1 2 2 2
  spline S116 degree 2 poles (47.7604, -3.5087) (47.7209, -3.4271) (47.5702, -3.3481) (47.4393, -3.3481) knots 0 0 0 1 2 2 2
  spline S117 degree 2 poles (47.4393, -3.3481) (47.3158, -3.3481) (47.0417, -3.5037) (46.9132, -3.6247) knots 0 0 0 1 2 2 2
  line L158 (46.9132, -3.6247) -> (46.9132, -5.334)
  line L159 (46.9132, -5.334) -> (46.5279, -5.334)
  line L160 (46.5279, -5.334) -> (46.5279, -3.0468)
  line L161 (46.5279, -3.0468) -> (46.9132, -3.0468)
  line L162 (46.9132, -3.0468) -> (46.9132, -3.2987)
  spline S118 degree 2 poles (46.9132, -3.2987) (47.0639, -3.148) (47.3603, -2.9825) (47.5381, -2.9825) knots 0 0 0 1 2 2 2
  spline S119 degree 2 poles (47.5381, -2.9825) (47.7407, -2.9825) (48.0544, -3.1678) (48.1359, -3.3777) knots 0 0 0 1 2 2 2
  spline S120 degree 2 poles (48.1359, -3.3777) (48.3113, -3.1826) (48.6422, -2.9825) (48.8349, -2.9825) knots 0 0 0 1 2 2 2
  spline S121 degree 2 poles (48.8349, -2.9825) (48.9831, -2.9825) (49.2252, -3.0739) (49.3141, -3.1777) knots 0 0 0 1 2 2 2
  spline S122 degree 2 poles (49.3141, -3.1777) (49.4055, -3.2814) (49.5067, -3.5926) (49.5067, -3.8273) knots 0 0 0 1 2 2 2
  line L163 (49.5067, -3.8273) -> (49.5067, -5.334)
  line L164 (49.5067, -5.334) -> (49.1214, -5.334)
  line L165 (-51.132, -36.1546) -> (-51.4951, -36.1546)
  line L166 (-51.4951, -36.1546) -> (-51.4951, -37.2019)
  line L167 (-51.4951, -37.2019) -> (-51.8878, -37.2019)
  line L168 (-51.8878, -37.2019) -> (-51.8878, -36.1546)
  line L169 (-51.8878, -36.1546) -> (-53.234, -36.1546)
  line L170 (-53.234, -36.1546) -> (-53.234, -35.7248)
  line L171 (-53.234, -35.7248) -> (-51.8705, -34.1539)
  line L172 (-51.8705, -34.1539) -> (-51.4951, -34.1539)
  line L173 (-51.4951, -34.1539) -> (-51.4951, -35.8261)
  line L174 (-51.4951, -35.8261) -> (-51.132, -35.8261)
  line L175 (-51.132, -35.8261) -> (-51.132, -36.1546)
  line L176 (-51.8878, -35.8261) -> (-51.8878, -34.6355)
  line L177 (-51.8878, -34.6355) -> (-52.9129, -35.8261)
  line L178 (-52.9129, -35.8261) -> (-51.8878, -35.8261)
  line L179 (-46.8465, -37.2019) -> (-46.8465, -35.8779)
  spline S123 degree 2 poles (-46.8465, -35.8779) (-46.8465, -35.7199) (-46.8712, -35.4506) (-46.9107, -35.3765) knots 0 0 0 1 2 2 2
  spline S124 degree 2 poles (-46.9107, -35.3765) (-46.9502, -35.295) (-47.1009, -35.216) (-47.2318, -35.216) knots 0 0 0 1 2 2 2
  spline S125 degree 2 poles (-47.2318, -35.216) (-47.3504, -35.216) (-47.6221, -35.3617) (-47.7654, -35.5) knots 0 0 0 1 2 2 2
  spline S126 degree 2 poles (-47.7654, -35.5) (-47.7629, -35.5346) (-47.7579, -35.6309) (-47.7579, -35.6952) knots 0 0 0 1 2 2 2
  line L180 (-47.7579, -35.6952) -> (-47.7579, -37.2019)
  line L181 (-47.7579, -37.2019) -> (-48.1433, -37.2019)
  line L182 (-48.1433, -37.2019) -> (-48.1433, -35.8779)
  spline S127 degree 2 poles (-48.1433, -35.8779) (-48.1433, -35.7199) (-48.168, -35.4506) (-48.2075, -35.3765) knots 0 0 0 1 2 2 2
  spline S128 degree 2 poles (-48.2075, -35.3765) (-48.247, -35.295) (-48.3977, -35.216) (-48.5286, -35.216) knots 0 0 0 1 2 2 2
  spline S129 degree 2 poles (-48.5286, -35.216) (-48.6521, -35.216) (-48.9263, -35.3716) (-49.0547, -35.4926) knots 0 0 0 1 2 2 2
  line L183 (-49.0547, -35.4926) -> (-49.0547, -37.2019)
  line L184 (-49.0547, -37.2019) -> (-49.44, -37.2019)
  line L185 (-49.44, -37.2019) -> (-49.44, -34.9146)
  line L186 (-49.44, -34.9146) -> (-49.0547, -34.9146)
  line L187 (-49.0547, -34.9146) -> (-49.0547, -35.1666)
  spline S130 degree 2 poles (-49.0547, -35.1666) (-48.904, -35.0159) (-48.6076, -34.8504) (-48.4298, -34.8504) knots 0 0 0 1 2 2 2
  spline S131 degree 2 poles (-48.4298, -34.8504) (-48.2272, -34.8504) (-47.9136, -35.0357) (-47.832, -35.2456) knots 0 0 0 1 2 2 2
  spline S132 degree 2 poles (-47.832, -35.2456) (-47.6567, -35.0505) (-47.3257, -34.8504) (-47.133, -34.8504) knots 0 0 0 1 2 2 2
  spline S133 degree 2 poles (-47.133, -34.8504) (-46.9848, -34.8504) (-46.7428, -34.9418) (-46.6538, -35.0455) knots 0 0 0 1 2 2 2
  spline S134 degree 2 poles (-46.6538, -35.0455) (-46.5625, -35.1493) (-46.4612, -35.4605) (-46.4612, -35.6952) knots 0 0 0 1 2 2 2
  line L188 (-46.4612, -35.6952) -> (-46.4612, -37.2019)
  line L189 (-46.4612, -37.2019) -> (-46.8465, -37.2019)
  line L190 (-43.3267, -37.2019) -> (-43.3267, -35.8779)
  spline S135 degree 2 poles (-43.3267, -35.8779) (-43.3267, -35.7199) (-43.3514, -35.4506) (-43.391, -35.3765) knots 0 0 0 1 2 2 2
  spline S136 degree 2 poles (-43.391, -35.3765) (-43.4305, -35.295) (-43.5811, -35.216) (-43.7121, -35.216) knots 0 0 0 1 2 2 2
  spline S137 degree 2 poles (-43.7121, -35.216) (-43.8306, -35.216) (-44.1023, -35.3617) (-44.2456, -35.5) knots 0 0 0 1 2 2 2
  spline S138 degree 2 poles (-44.2456, -35.5) (-44.2431, -35.5346) (-44.2382, -35.6309) (-44.2382, -35.6952) knots 0 0 0 1 2 2 2
  line L191 (-44.2382, -35.6952) -> (-44.2382, -37.2019)
  line L192 (-44.2382, -37.2019) -> (-44.6235, -37.2019)
  line L193 (-44.6235, -37.2019) -> (-44.6235, -35.8779)
  spline S139 degree 2 poles (-44.6235, -35.8779) (-44.6235, -35.7199) (-44.6482, -35.4506) (-44.6877, -35.3765) knots 0 0 0 1 2 2 2
  spline S140 degree 2 poles (-44.6877, -35.3765) (-44.7272, -35.295) (-44.8779, -35.216) (-45.0088, -35.216) knots 0 0 0 1 2 2 2
  spline S141 degree 2 poles (-45.0088, -35.216) (-45.1323, -35.216) (-45.4065, -35.3716) (-45.5349, -35.4926) knots 0 0 0 1 2 2 2
  line L194 (-45.5349, -35.4926) -> (-45.5349, -37.2019)
  line L195 (-45.5349, -37.2019) -> (-45.9202, -37.2019)
  line L196 (-45.9202, -37.2019) -> (-45.9202, -34.9146)
  line L197 (-45.9202, -34.9146) -> (-45.5349, -34.9146)
  line L198 (-45.5349, -34.9146) -> (-45.5349, -35.1666)
  spline S142 degree 2 poles (-45.5349, -35.1666) (-45.3843, -35.0159) (-45.0879, -34.8504) (-44.91, -34.8504) knots 0 0 0 1 2 2 2
  spline S143 degree 2 poles (-44.91, -34.8504) (-44.7075, -34.8504) (-44.3938, -35.0357) (-44.3123, -35.2456) knots 0 0 0 1 2 2 2
  spline S144 degree 2 poles (-44.3123, -35.2456) (-44.1369, -35.0505) (-43.8059, -34.8504) (-43.6133, -34.8504) knots 0 0 0 1 2 2 2
  spline S145 degree 2 poles (-43.6133, -34.8504) (-43.4651, -34.8504) (-43.223, -34.9418) (-43.1341, -35.0455) knots 0 0 0 1 2 2 2
  spline S146 degree 2 poles (-43.1341, -35.0455) (-43.0427, -35.1493) (-42.9414, -35.4605) (-42.9414, -35.6952) knots 0 0 0 1 2 2 2
  line L199 (-42.9414, -35.6952) -> (-42.9414, -37.2019)
  line L200 (-42.9414, -37.2019) -> (-43.3267, -37.2019)
  spline S147 degree 2 poles (-28.1231, -36.2336) (-28.1231, -36.4535) (-28.2639, -36.8289) (-28.3924, -36.9672) knots 0 0 0 1 2 2 2
  spline S148 degree 2 poles (-28.3924, -36.9672) (-28.5208, -37.1055) (-28.9037, -37.2661) (-29.1408, -37.2661) knots 0 0 0 1 2 2 2
  spline S149 degree 2 poles (-29.1408, -37.2661) (-29.3581, -37.2661) (-29.783, -37.1698) (-29.9386, -37.0932) knots 0 0 0 1 2 2 2
  line L201 (-29.9386, -37.0932) -> (-29.9386, -36.6609)
  line L202 (-29.9386, -36.6609) -> (-29.909, -36.6609)
  spline S150 degree 2 poles (-29.909, -36.6609) (-29.862, -36.6955) (-29.6867, -36.7844) (-29.5804, -36.824) knots 0 0 0 1 2 2 2
  spline S151 degree 2 poles (-29.5804, -36.824) (-29.4594, -36.8659) (-29.2593, -36.9129) (-29.1334, -36.9129) knots 0 0 0 1 2 2 2
  spline S152 degree 2 poles (-29.1334, -36.9129) (-29.0099, -36.9129) (-28.7777, -36.824) (-28.6937, -36.7276) knots 0 0 0 1 2 2 2
  spline S153 degree 2 poles (-28.6937, -36.7276) (-28.6171, -36.6362) (-28.5381, -36.3942) (-28.5381, -36.2312) knots 0 0 0 1 2 2 2
  spline S154 degree 2 poles (-28.5381, -36.2312) (-28.5381, -36.0681) (-28.627, -35.8606) (-28.711, -35.7915) knots 0 0 0 1 2 2 2
  spline S155 degree 2 poles (-28.711, -35.7915) (-28.7975, -35.7149) (-29.0543, -35.6507) (-29.2099, -35.6507) knots 0 0 0 1 2 2 2
  spline S156 degree 2 poles (-29.2099, -35.6507) (-29.3779, -35.6507) (-29.7114, -35.7026) (-29.8126, -35.7248) knots 0 0 0 1 2 2 2
  line L203 (-29.8126, -35.7248) -> (-29.8126, -34.1539)
  line L204 (-29.8126, -34.1539) -> (-28.1404, -34.1539)
  line L205 (-28.1404, -34.1539) -> (-28.1404, -34.512)
  line L206 (-28.1404, -34.512) -> (-29.4199, -34.512)
  line L207 (-29.4199, -34.512) -> (-29.4199, -35.3247)
  spline S157 degree 2 poles (-29.4199, -35.3247) (-29.3458, -35.3148) (-29.2025, -35.3074) (-29.1433, -35.3074) knots 0 0 0 1 2 2 2
  spline S158 degree 2 poles (-29.1433, -35.3074) (-28.9086, -35.3074) (-28.585, -35.3839) (-28.4368, -35.4976) knots 0 0 0 1 2 2 2
  spline S159 degree 2 poles (-28.4368, -35.4976) (-28.2862, -35.6112) (-28.1231, -35.957) (-28.1231, -36.2336) knots 0 0 0 1 2 2 2
  line L208 (-23.724, -37.2019) -> (-23.724, -35.8779)
  spline S160 degree 2 poles (-23.724, -35.8779) (-23.724, -35.7199) (-23.7487, -35.4506) (-23.7883, -35.3765) knots 0 0 0 1 2 2 2
  spline S161 degree 2 poles (-23.7883, -35.3765) (-23.8278, -35.295) (-23.9785, -35.216) (-24.1094, -35.216) knots 0 0 0 1 2 2 2
  spline S162 degree 2 poles (-24.1094, -35.216) (-24.2279, -35.216) (-24.4996, -35.3617) (-24.6429, -35.5) knots 0 0 0 1 2 2 2
  spline S163 degree 2 poles (-24.6429, -35.5) (-24.6404, -35.5346) (-24.6355, -35.6309) (-24.6355, -35.6952) knots 0 0 0 1 2 2 2
  line L209 (-24.6355, -35.6952) -> (-24.6355, -37.2019)
  line L210 (-24.6355, -37.2019) -> (-25.0208, -37.2019)
  line L211 (-25.0208, -37.2019) -> (-25.0208, -35.8779)
  spline S164 degree 2 poles (-25.0208, -35.8779) (-25.0208, -35.7199) (-25.0455, -35.4506) (-25.085, -35.3765) knots 0 0 0 1 2 2 2
  spline S165 degree 2 poles (-25.085, -35.3765) (-25.1245, -35.295) (-25.2752, -35.216) (-25.4061, -35.216) knots 0 0 0 1 2 2 2
  spline S166 degree 2 poles (-25.4061, -35.216) (-25.5296, -35.216) (-25.8038, -35.3716) (-25.9322, -35.4926) knots 0 0 0 1 2 2 2
  line L212 (-25.9322, -35.4926) -> (-25.9322, -37.2019)
  line L213 (-25.9322, -37.2019) -> (-26.3176, -37.2019)
  line L214 (-26.3176, -37.2019) -> (-26.3176, -34.9146)
  line L215 (-26.3176, -34.9146) -> (-25.9322, -34.9146)
  line L216 (-25.9322, -34.9146) -> (-25.9322, -35.1666)
  spline S167 degree 2 poles (-25.9322, -35.1666) (-25.7816, -35.0159) (-25.4852, -34.8504) (-25.3073, -34.8504) knots 0 0 0 1 2 2 2
  spline S168 degree 2 poles (-25.3073, -34.8504) (-25.1048, -34.8504) (-24.7911, -35.0357) (-24.7096, -35.2456) knots 0 0 0 1 2 2 2
  spline S169 degree 2 poles (-24.7096, -35.2456) (-24.5342, -35.0505) (-24.2032, -34.8504) (-24.0106, -34.8504) knots 0 0 0 1 2 2 2
  spline S170 degree 2 poles (-24.0106, -34.8504) (-23.8624, -34.8504) (-23.6203, -34.9418) (-23.5314, -35.0455) knots 0 0 0 1 2 2 2
  spline S171 degree 2 poles (-23.5314, -35.0455) (-23.44, -35.1493) (-23.3387, -35.4605) (-23.3387, -35.6952) knots 0 0 0 1 2 2 2
  line L217 (-23.3387, -35.6952) -> (-23.3387, -37.2019)
  line L218 (-23.3387, -37.2019) -> (-23.724, -37.2019)
  line L219 (-20.2043, -37.2019) -> (-20.2043, -35.8779)
  spline S172 degree 2 poles (-20.2043, -35.8779) (-20.2043, -35.7199) (-20.229, -35.4506) (-20.2685, -35.3765) knots 0 0 0 1 2 2 2
  spline S173 degree 2 poles (-20.2685, -35.3765) (-20.308, -35.295) (-20.4587, -35.216) (-20.5896, -35.216) knots 0 0 0 1 2 2 2
  spline S174 degree 2 poles (-20.5896, -35.216) (-20.7081, -35.216) (-20.9799, -35.3617) (-21.1231, -35.5) knots 0 0 0 1 2 2 2
  spline S175 degree 2 poles (-21.1231, -35.5) (-21.1206, -35.5346) (-21.1157, -35.6309) (-21.1157, -35.6952) knots 0 0 0 1 2 2 2
  line L220 (-21.1157, -35.6952) -> (-21.1157, -37.2019)
  line L221 (-21.1157, -37.2019) -> (-21.501, -37.2019)
  line L222 (-21.501, -37.2019) -> (-21.501, -35.8779)
  spline S176 degree 2 poles (-21.501, -35.8779) (-21.501, -35.7199) (-21.5257, -35.4506) (-21.5652, -35.3765) knots 0 0 0 1 2 2 2
  spline S177 degree 2 poles (-21.5652, -35.3765) (-21.6048, -35.295) (-21.7554, -35.216) (-21.8863, -35.216) knots 0 0 0 1 2 2 2
  spline S178 degree 2 poles (-21.8863, -35.216) (-22.0098, -35.216) (-22.284, -35.3716) (-22.4125, -35.4926) knots 0 0 0 1 2 2 2
  line L223 (-22.4125, -35.4926) -> (-22.4125, -37.2019)
  line L224 (-22.4125, -37.2019) -> (-22.7978, -37.2019)
  line L225 (-22.7978, -37.2019) -> (-22.7978, -34.9146)
  line L226 (-22.7978, -34.9146) -> (-22.4125, -34.9146)
  line L227 (-22.4125, -34.9146) -> (-22.4125, -35.1666)
  spline S179 degree 2 poles (-22.4125, -35.1666) (-22.2618, -35.0159) (-21.9654, -34.8504) (-21.7875, -34.8504) knots 0 0 0 1 2 2 2
  spline S180 degree 2 poles (-21.7875, -34.8504) (-21.585, -34.8504) (-21.2713, -35.0357) (-21.1898, -35.2456) knots 0 0 0 1 2 2 2
  spline S181 degree 2 poles (-21.1898, -35.2456) (-21.0144, -35.0505) (-20.6834, -34.8504) (-20.4908, -34.8504) knots 0 0 0 1 2 2 2
  spline S182 degree 2 poles (-20.4908, -34.8504) (-20.3426, -34.8504) (-20.1005, -34.9418) (-20.0116, -35.0455) knots 0 0 0 1 2 2 2
  spline S183 degree 2 poles (-20.0116, -35.0455) (-19.9202, -35.1493) (-19.8189, -35.4605) (-19.8189, -35.6952) knots 0 0 0 1 2 2 2
  line L228 (-19.8189, -35.6952) -> (-19.8189, -37.2019)
  line L229 (-19.8189, -37.2019) -> (-20.2043, -37.2019)
  spline S184 degree 2 poles (-4.9216, -36.2139) (-4.9216, -36.4485) (-5.0772, -36.8462) (-5.2082, -36.9796) knots 0 0 0 1 2 2 2
  spline S185 degree 2 poles (-5.2082, -36.9796) (-5.344, -37.1204) (-5.6849, -37.2661) (-5.8899, -37.2661) knots 0 0 0 1 2 2 2
  spline S186 degree 2 poles (-5.8899, -37.2661) (-6.0949, -37.2661) (-6.4333, -37.1278) (-6.5617, -36.9894) knots 0 0 0 1 2 2 2
  spline S187 degree 2 poles (-6.5617, -36.9894) (-6.7198, -36.824) (-6.8976, -36.2682) (-6.8976, -35.8631) knots 0 0 0 1 2 2 2
  spline S188 degree 2 poles (-6.8976, -35.8631) (-6.8976, -35.4654) (-6.7346, -34.8257) (-6.5642, -34.5886) knots 0 0 0 1 2 2 2
  spline S189 degree 2 poles (-6.5642, -34.5886) (-6.3987, -34.3564) (-5.8751, -34.0971) (-5.5317, -34.0971) knots 0 0 0 1 2 2 2
  spline S190 degree 2 poles (-5.5317, -34.0971) (-5.4305, -34.0971) (-5.2526, -34.1168) (-5.1859, -34.139) knots 0 0 0 1 2 2 2
  line L230 (-5.1859, -34.139) -> (-5.1859, -34.5318)
  line L231 (-5.1859, -34.5318) -> (-5.2032, -34.5318)
  spline S191 degree 2 poles (-5.2032, -34.5318) (-5.26, -34.5021) (-5.4675, -34.4503) (-5.5861, -34.4503) knots 0 0 0 1 2 2 2
  spline S192 degree 2 poles (-5.5861, -34.4503) (-5.9664, -34.4503) (-6.4333, -34.964) (-6.4777, -35.4679) knots 0 0 0 1 2 2 2
  spline S193 degree 2 poles (-6.4777, -35.4679) (-6.332, -35.3666) (-6.0257, -35.2555) (-5.8429, -35.2555) knots 0 0 0 1 2 2 2
  spline S194 degree 2 poles (-5.8429, -35.2555) (-5.6651, -35.2555) (-5.3983, -35.3271) (-5.2526, -35.4358) knots 0 0 0 1 2 2 2
  spline S195 degree 2 poles (-5.2526, -35.4358) (-5.0847, -35.5618) (-4.9216, -35.952) (-4.9216, -36.2139) knots 0 0 0 1 2 2 2
  spline S196 degree 2 poles (-5.3366, -36.2312) (-5.3366, -36.0434) (-5.4354, -35.789) (-5.5441, -35.7001) knots 0 0 0 1 2 2 2
  spline S197 degree 2 poles (-5.5441, -35.7001) (-5.6256, -35.6359) (-5.8281, -35.5939) (-5.9343, -35.5939) knots 0 0 0 1 2 2 2
  spline S198 degree 2 poles (-5.9343, -35.5939) (-6.0776, -35.5939) (-6.3468, -35.6803) (-6.4777, -35.7618) knots 0 0 0 1 2 2 2
  spline S199 degree 2 poles (-6.4777, -35.7618) (-6.4802, -35.8063) (-6.4852, -35.8903) (-6.4852, -35.9545) knots 0 0 0 1 2 2 2
  spline S200 degree 2 poles (-6.4852, -35.9545) (-6.4852, -36.2707) (-6.3617, -36.6585) (-6.2678, -36.7597) knots 0 0 0 1 2 2 2
  spline S201 degree 2 poles (-6.2678, -36.7597) (-6.1813, -36.8561) (-5.9936, -36.9326) (-5.8874, -36.9326) knots 0 0 0 1 2 2 2
  spline S202 degree 2 poles (-5.8874, -36.9326) (-5.6404, -36.9326) (-5.3366, -36.5819) (-5.3366, -36.2312) knots 0 0 0 1 2 2 2
  line L232 (-0.6016, -37.2019) -> (-0.6016, -35.8779)
  spline S203 degree 2 poles (-0.6016, -35.8779) (-0.6016, -35.7199) (-0.6263, -35.4506) (-0.6658, -35.3765) knots 0 0 0 1 2 2 2
  spline S204 degree 2 poles (-0.6658, -35.3765) (-0.7053, -35.295) (-0.856, -35.216) (-0.9869, -35.216) knots 0 0 0 1 2 2 2
  spline S205 degree 2 poles (-0.9869, -35.216) (-1.1055, -35.216) (-1.3772, -35.3617) (-1.5204, -35.5) knots 0 0 0 1 2 2 2
  spline S206 degree 2 poles (-1.5204, -35.5) (-1.5179, -35.5346) (-1.513, -35.6309) (-1.513, -35.6952) knots 0 0 0 1 2 2 2
  line L233 (-1.513, -35.6952) -> (-1.513, -37.2019)
  line L234 (-1.513, -37.2019) -> (-1.8983, -37.2019)
  line L235 (-1.8983, -37.2019) -> (-1.8983, -35.8779)
  spline S207 degree 2 poles (-1.8983, -35.8779) (-1.8983, -35.7199) (-1.923, -35.4506) (-1.9626, -35.3765) knots 0 0 0 1 2 2 2
  spline S208 degree 2 poles (-1.9626, -35.3765) (-2.0021, -35.295) (-2.1527, -35.216) (-2.2837, -35.216) knots 0 0 0 1 2 2 2
  spline S209 degree 2 poles (-2.2837, -35.216) (-2.4072, -35.216) (-2.6813, -35.3716) (-2.8098, -35.4926) knots 0 0 0 1 2 2 2
  line L236 (-2.8098, -35.4926) -> (-2.8098, -37.2019)
  line L237 (-2.8098, -37.2019) -> (-3.1951, -37.2019)
  line L238 (-3.1951, -37.2019) -> (-3.1951, -34.9146)
  line L239 (-3.1951, -34.9146) -> (-2.8098, -34.9146)
  line L240 (-2.8098, -34.9146) -> (-2.8098, -35.1666)
  spline S210 degree 2 poles (-2.8098, -35.1666) (-2.6591, -35.0159) (-2.3627, -34.8504) (-2.1849, -34.8504) knots 0 0 0 1 2 2 2
  spline S211 degree 2 poles (-2.1849, -34.8504) (-1.9823, -34.8504) (-1.6686, -35.0357) (-1.5871, -35.2456) knots 0 0 0 1 2 2 2
  spline S212 degree 2 poles (-1.5871, -35.2456) (-1.4117, -35.0505) (-1.0808, -34.8504) (-0.8881, -34.8504) knots 0 0 0 1 2 2 2
  spline S213 degree 2 poles (-0.8881, -34.8504) (-0.7399, -34.8504) (-0.4978, -34.9418) (-0.4089, -35.0455) knots 0 0 0 1 2 2 2
  spline S214 degree 2 poles (-0.4089, -35.0455) (-0.3175, -35.1493) (-0.2162, -35.4605) (-0.2162, -35.6952) knots 0 0 0 1 2 2 2
  line L241 (-0.2162, -35.6952) -> (-0.2162, -37.2019)
  line L242 (-0.2162, -37.2019) -> (-0.6016, -37.2019)
  line L243 (2.9182, -37.2019) -> (2.9182, -35.8779)
  spline S215 degree 2 poles (2.9182, -35.8779) (2.9182, -35.7199) (2.8935, -35.4506) (2.854, -35.3765) knots 0 0 0 1 2 2 2
  spline S216 degree 2 poles (2.854, -35.3765) (2.8145, -35.295) (2.6638, -35.216) (2.5329, -35.216) knots 0 0 0 1 2 2 2
  spline S217 degree 2 poles (2.5329, -35.216) (2.4143, -35.216) (2.1426, -35.3617) (1.9994, -35.5) knots 0 0 0 1 2 2 2
  spline S218 degree 2 poles (1.9994, -35.5) (2.0018, -35.5346) (2.0068, -35.6309) (2.0068, -35.6952) knots 0 0 0 1 2 2 2
  line L244 (2.0068, -35.6952) -> (2.0068, -37.2019)
  line L245 (2.0068, -37.2019) -> (1.6214, -37.2019)
  line L246 (1.6214, -37.2019) -> (1.6214, -35.8779)
  spline S219 degree 2 poles (1.6214, -35.8779) (1.6214, -35.7199) (1.5967, -35.4506) (1.5572, -35.3765) knots 0 0 0 1 2 2 2
  spline S220 degree 2 poles (1.5572, -35.3765) (1.5177, -35.295) (1.367, -35.216) (1.2361, -35.216) knots 0 0 0 1 2 2 2
  spline S221 degree 2 poles (1.2361, -35.216) (1.1126, -35.216) (0.8384, -35.3716) (0.71, -35.4926) knots 0 0 0 1 2 2 2
  line L247 (0.71, -35.4926) -> (0.71, -37.2019)
  line L248 (0.71, -37.2019) -> (0.3247, -37.2019)
  line L249 (0.3247, -37.2019) -> (0.3247, -34.9146)
  line L250 (0.3247, -34.9146) -> (0.71, -34.9146)
  line L251 (0.71, -34.9146) -> (0.71, -35.1666)
  spline S222 degree 2 poles (0.71, -35.1666) (0.8607, -35.0159) (1.1571, -34.8504) (1.3349, -34.8504) knots 0 0 0 1 2 2 2
  spline S223 degree 2 poles (1.3349, -34.8504) (1.5375, -34.8504) (1.8512, -35.0357) (1.9327, -35.2456) knots 0 0 0 1 2 2 2
  spline S224 degree 2 poles (1.9327, -35.2456) (2.108, -35.0505) (2.439, -34.8504) (2.6317, -34.8504) knots 0 0 0 1 2 2 2
  spline S225 degree 2 poles (2.6317, -34.8504) (2.7799, -34.8504) (3.0219, -34.9418) (3.1109, -35.0455) knots 0 0 0 1 2 2 2
  spline S226 degree 2 poles (3.1109, -35.0455) (3.2023, -35.1493) (3.3035, -35.4605) (3.3035, -35.6952) knots 0 0 0 1 2 2 2
  line L252 (3.3035, -35.6952) -> (3.3035, -37.2019)
  line L253 (3.3035, -37.2019) -> (2.9182, -37.2019)
  line L254 (19.0775, -34.6108) -> (17.7585, -37.2019)
  line L255 (17.7585, -37.2019) -> (17.3238, -37.2019)
  line L256 (17.3238, -37.2019) -> (18.7169, -34.512)
  line L257 (18.7169, -34.512) -> (17.1435, -34.512)
  line L258 (17.1435, -34.512) -> (17.1435, -34.1539)
  line L259 (17.1435, -34.1539) -> (19.0775, -34.1539)
  line L260 (19.0775, -34.1539) -> (19.0775, -34.6108)
  line L261 (23.4099, -37.2019) -> (23.4099, -35.8779)
  spline S227 degree 2 poles (23.4099, -35.8779) (23.4099, -35.7199) (23.3852, -35.4506) (23.3457, -35.3765) knots 0 0 0 1 2 2 2
  spline S228 degree 2 poles (23.3457, -35.3765) (23.3062, -35.295) (23.1555, -35.216) (23.0246, -35.216) knots 0 0 0 1 2 2 2
  spline S229 degree 2 poles (23.0246, -35.216) (22.906, -35.216) (22.6343, -35.3617) (22.491, -35.5) knots 0 0 0 1 2 2 2
  spline S230 degree 2 poles (22.491, -35.5) (22.4935, -35.5346) (22.4985, -35.6309) (22.4985, -35.6952) knots 0 0 0 1 2 2 2
  line L262 (22.4985, -35.6952) -> (22.4985, -37.2019)
  line L263 (22.4985, -37.2019) -> (22.1131, -37.2019)
  line L264 (22.1131, -37.2019) -> (22.1131, -35.8779)
  spline S231 degree 2 poles (22.1131, -35.8779) (22.1131, -35.7199) (22.0884, -35.4506) (22.0489, -35.3765) knots 0 0 0 1 2 2 2
  spline S232 degree 2 poles (22.0489, -35.3765) (22.0094, -35.295) (21.8587, -35.216) (21.7278, -35.216) knots 0 0 0 1 2 2 2
  spline S233 degree 2 poles (21.7278, -35.216) (21.6043, -35.216) (21.3301, -35.3716) (21.2017, -35.4926) knots 0 0 0 1 2 2 2
  line L265 (21.2017, -35.4926) -> (21.2017, -37.2019)
  line L266 (21.2017, -37.2019) -> (20.8164, -37.2019)
  line L267 (20.8164, -37.2019) -> (20.8164, -34.9146)
  line L268 (20.8164, -34.9146) -> (21.2017, -34.9146)
  line L269 (21.2017, -34.9146) -> (21.2017, -35.1666)
  spline S234 degree 2 poles (21.2017, -35.1666) (21.3524, -35.0159) (21.6488, -34.8504) (21.8266, -34.8504) knots 0 0 0 1 2 2 2
  spline S235 degree 2 poles (21.8266, -34.8504) (22.0292, -34.8504) (22.3428, -35.0357) (22.4244, -35.2456) knots 0 0 0 1 2 2 2
  spline S236 degree 2 poles (22.4244, -35.2456) (22.5997, -35.0505) (22.9307, -34.8504) (23.1234, -34.8504) knots 0 0 0 1 2 2 2
  spline S237 degree 2 poles (23.1234, -34.8504) (23.2716, -34.8504) (23.5136, -34.9418) (23.6026, -35.0455) knots 0 0 0 1 2 2 2
  spline S238 degree 2 poles (23.6026, -35.0455) (23.6939, -35.1493) (23.7952, -35.4605) (23.7952, -35.6952) knots 0 0 0 1 2 2 2
  line L270 (23.7952, -35.6952) -> (23.7952, -37.2019)
  line L271 (23.7952, -37.2019) -> (23.4099, -37.2019)
  line L272 (26.9297, -37.2019) -> (26.9297, -35.8779)
  spline S239 degree 2 poles (26.9297, -35.8779) (26.9297, -35.7199) (26.905, -35.4506) (26.8654, -35.3765) knots 0 0 0 1 2 2 2
  spline S240 degree 2 poles (26.8654, -35.3765) (26.8259, -35.295) (26.6753, -35.216) (26.5443, -35.216) knots 0 0 0 1 2 2 2
  spline S241 degree 2 poles (26.5443, -35.216) (26.4258, -35.216) (26.1541, -35.3617) (26.0108, -35.5) knots 0 0 0 1 2 2 2
  spline S242 degree 2 poles (26.0108, -35.5) (26.0133, -35.5346) (26.0182, -35.6309) (26.0182, -35.6952) knots 0 0 0 1 2 2 2
  line L273 (26.0182, -35.6952) -> (26.0182, -37.2019)
  line L274 (26.0182, -37.2019) -> (25.6329, -37.2019)
  line L275 (25.6329, -37.2019) -> (25.6329, -35.8779)
  spline S243 degree 2 poles (25.6329, -35.8779) (25.6329, -35.7199) (25.6082, -35.4506) (25.5687, -35.3765) knots 0 0 0 1 2 2 2